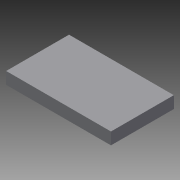
# Autodesk Inventor part: Ceramic Heating Element
Saved by Autodesk Inventor 2015 (Build 190159000, 159)
## iProperties
Created: 2016-08-07
Part Number: Ceramic Heating Element
Material: Generic
Document SubType Name: Modeling
Designer: spichelh
Density: 1 g/cm^3
Appearance: Default
Author: spichelh
Autodesk Inventor part; units mm, degrees
ref_plane "YZ Plane" through (0, 0, 0) normal (1, 0, 0) x (0, 1, 0)
ref_plane "XZ Plane" through (0, 0, 0) normal (0, 1, 0) x (-1, 0, 0)
ref_plane "XY Plane" through (0, 0, 0) normal (0, 0, 1) x (1, 0, 0)
sketch "Sketch1" plane through (0, 0, 0) normal (0, 1, 0) x (-1, 0, 0)
  line L0 (0, 0) -> (-35, 0)
  line L1 (-35, 0) -> (-35, -21)
  line L2 (-35, -21) -> (0, -21)
  line L3 (0, -21) -> (0, 0)
  dimension "d0" = 35
  dimension "d1" = 21
  constraints: 8 end point, 2 parallel, 1 horizontal, 1 perpendicular
  measures "d0" distance of L1.end L2.end
  measures "d1" distance between parallel lines of L0 L2
extrude "Extrusion1" add sketch "Sketch1" along normal blind 4
body "Solid1"
